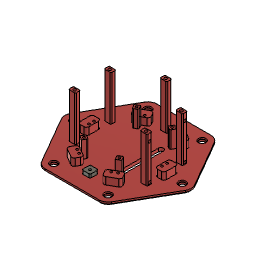
2024-12-28_development_hexapod_mounts (Autodesk Fusion 360 archive; units mm, degrees)
design "base"
Autodesk Fusion 360 part; units mm, degrees
(part 1 of 2)
sketch "Sketch1" plane through (0, 0, 0) normal (0, 0, 1) x (1, 0, 0)
  line L0 (130, 0) -> (65, 112.5833)
  line L1 (65, 112.5833) -> (-65, 112.5833)
  line L2 (-65, 112.5833) -> (-130, 0)
  line L3 (-130, 0) -> (-65, -112.5833)
  line L4 (-65, -112.5833) -> (65, -112.5833)
  line L5 (65, -112.5833) -> (130, 0)
  dimension "d1" = 130
  measures "d1" distance of L0.start origin
extrude "Extrude1" add sketch "Sketch1" along normal blind 6.5 makes body 1
fillet "Fillet1" radius 18 6 edges at (-130, 0, 3.25) (-65, -112.5833, 3.25) (65, -112.5833, 3.25) (130, 0, 3.25) (65, 112.5833, 3.25) (-65, 112.5833, 3.25) on bodies 1
chamfer "Chamfer2" distance 3.25 angle 45 12 edges at (0, -112.5833, 0) (63.6077, -110.1718, 0) (97.5, -56.2917, 0) (127.2154, 0, 0) (97.5, 56.2917, 0) (63.6077, 110.1718, 0) (0, 112.5833, 0) (-63.6077, 110.1718, 0) (-97.5, 56.2917, 0) (-127.2154, 0, 0) (-97.5, -56.2917, 0) (-63.6077, -110.1718, 0) on bodies 1
sketch "Sketch2" plane through (0, 0, 6.5) normal (0, 0, 1) x (-1, 0, 0)
  arc A0 (54.6077, -112.5833) -> (70.1962, -103.5833) centre (54.6077, -94.5833) ccw
  line L0 (70.1962, -103.5833) -> (124.8038, -9)
  arc A1 (124.8038, -9) -> (124.8038, 9) centre (109.2154, 0) ccw
  line L1 (124.8038, 9) -> (70.1962, 103.5833)
  line L2 (54.6077, 112.5833) -> (-54.6077, 112.5833)
  line L3 (-70.1962, 103.5833) -> (-124.8038, 9)
  arc A2 (-124.8038, 9) -> (-124.8038, -9) centre (-109.2154, 0) ccw
  line L4 (-124.8038, -9) -> (-70.1962, -103.5833)
  arc A3 (-70.1962, -103.5833) -> (-54.6077, -112.5833) centre (-54.6077, -94.5833) ccw
  line L5 (-54.6077, -112.5833) -> (54.6077, -112.5833)
  circle A4 centre (109.2154, 0) radius 7
  circle A5 centre (109.2154, 0) radius 6
  circle A6 centre (73.4654, -5) radius 2.25
  arc A7 (73.7154, 14.55) -> (68.7154, 9.55) centre (73.7154, 9.55) ccw
  line L6 (68.7154, 9.55) -> (68.7154, -9.55)
  circle A8 centre (73.4654, 5) radius 2.25
  line L7 (86.7154, 9.55) -> (86.7154, -9.55)
  line L8 (68.7154, 0) -> (86.7154, 0) construction
  arc A9 (68.7154, -9.55) -> (73.7154, -14.55) centre (73.7154, -9.55) ccw
  arc A10 (73.7154, 14.55) -> (68.7154, 9.55) centre (73.7154, 9.55) ccw
  line L9 (81.7154, 14.55) -> (73.7154, 14.55)
  line L10 (73.7154, -14.55) -> (81.7154, -14.55)
  line L11 (73.4654, 5) -> (68.7154, 5) construction
  line L12 (73.4654, -5) -> (68.7154, -5) construction
  line L13 (127.2154, 0) -> (-127.2154, 0) construction
  line L14 (0, -112.5833) -> (0, 112.5833) construction
  arc A11 (-124.8038, 9) -> (-124.8038, -9) centre (-109.2154, 0) ccw
  arc A12 (-70.1962, -103.5833) -> (-54.6077, -112.5833) centre (-54.6077, -94.5833) ccw
  arc A13 (54.6077, -112.5833) -> (70.1962, -103.5833) centre (54.6077, -94.5833) ccw
  arc A14 (81.7154, -14.55) -> (86.7154, -9.55) centre (81.7154, -9.55) ccw
  arc A15 (86.7154, 9.55) -> (81.7154, 14.55) centre (81.7154, 9.55) ccw
  circle A16 centre (32.4026, 66.1229) radius 2.25
  line L15 (34.3577, 59.5093) -> (43.3577, 75.0977) construction
  arc A17 (70.1962, 103.5833) -> (54.6077, 112.5833) centre (54.6077, 94.5833) ccw
  arc A18 (42.6282, 54.7343) -> (49.4584, 56.5644) centre (45.1282, 59.0644) ccw
  line L16 (41.0628, 61.1229) -> (38.6878, 57.0093) construction
  arc A19 (24.257, 71.1144) -> (26.0872, 64.2843) centre (28.5872, 68.6144) ccw
  line L17 (28.257, 78.0426) -> (24.257, 71.1144)
  circle A20 centre (41.0628, 61.1229) radius 2.25
  arc A21 (53.4584, 63.4926) -> (51.6282, 70.3227) centre (49.1282, 65.9926) ccw
  circle A22 centre (54.6077, 94.5833) radius 6
  circle A23 centre (54.6077, 94.5833) radius 7
  line L18 (32.4026, 66.1229) -> (30.0276, 62.0093) construction
  arc A24 (24.257, 71.1144) -> (26.0872, 64.2843) centre (28.5872, 68.6144) ccw
  line L19 (26.0872, 64.2843) -> (42.6282, 54.7343)
  line L20 (49.4584, 56.5644) -> (53.4584, 63.4926)
  line L21 (35.0872, 79.8727) -> (51.6282, 70.3227)
  arc A25 (35.0872, 79.8727) -> (28.257, 78.0426) centre (32.5872, 75.5426) ccw
  circle A26 centre (-41.0628, 61.1229) radius 2.25
  line L22 (-42.6282, 54.7343) -> (-26.0872, 64.2843)
  line L23 (-34.3577, 59.5093) -> (-43.3577, 75.0977) construction
  arc A27 (-54.6077, 112.5833) -> (-70.1962, 103.5833) centre (-54.6077, 94.5833) ccw
  arc A28 (-26.0872, 64.2843) -> (-24.257, 71.1144) centre (-28.5872, 68.6144) ccw
  line L24 (-32.4026, 66.1229) -> (-30.0276, 62.0093) construction
  arc A29 (-49.4584, 56.5644) -> (-42.6282, 54.7343) centre (-45.1282, 59.0644) ccw
  line L25 (-53.4584, 63.4926) -> (-49.4584, 56.5644)
  circle A30 centre (-32.4026, 66.1229) radius 2.25
  arc A31 (-28.257, 78.0426) -> (-35.0872, 79.8727) centre (-32.5872, 75.5426) ccw
  circle A32 centre (-54.6077, 94.5833) radius 6
  circle A33 centre (-54.6077, 94.5833) radius 7
  line L26 (-41.0628, 61.1229) -> (-38.6878, 57.0093) construction
  arc A34 (-49.4584, 56.5644) -> (-42.6282, 54.7343) centre (-45.1282, 59.0644) ccw
  line L27 (-42.6282, 54.7343) -> (-26.0872, 64.2843)
  line L28 (-24.257, 71.1144) -> (-28.257, 78.0426)
  line L29 (-51.6282, 70.3227) -> (-35.0872, 79.8727)
  arc A35 (-51.6282, 70.3227) -> (-53.4584, 63.4926) centre (-49.1282, 65.9926) ccw
  circle A36 centre (-73.4654, -5) radius 2.25
  line L30 (-68.7154, -9.55) -> (-68.7154, 9.55)
  line L31 (-68.7154, 0) -> (-86.7154, 0) construction
  arc A37 (-124.8038, 9) -> (-124.8038, -9) centre (-109.2154, 0) ccw
  arc A38 (-68.7154, 9.55) -> (-73.7154, 14.55) centre (-73.7154, 9.55) ccw
  line L32 (-73.4654, 5) -> (-68.7154, 5) construction
  arc A39 (-73.7154, -14.55) -> (-68.7154, -9.55) centre (-73.7154, -9.55) ccw
  line L33 (-81.7154, -14.55) -> (-73.7154, -14.55)
  circle A40 centre (-73.4654, 5) radius 2.25
  arc A41 (-81.7154, 14.55) -> (-86.7154, 9.55) centre (-81.7154, 9.55) ccw
  circle A42 centre (-109.2154, 0) radius 6
  circle A43 centre (-109.2154, 0) radius 7
  line L34 (-73.4654, -5) -> (-68.7154, -5) construction
  arc A44 (-73.7154, -14.55) -> (-68.7154, -9.55) centre (-73.7154, -9.55) ccw
  line L35 (-68.7154, -9.55) -> (-68.7154, 9.55)
  line L36 (-73.7154, 14.55) -> (-81.7154, 14.55)
  line L37 (-86.7154, -9.55) -> (-86.7154, 9.55)
  arc A45 (-86.7154, -9.55) -> (-81.7154, -14.55) centre (-81.7154, -9.55) ccw
  circle A46 centre (-32.4026, -66.1229) radius 2.25
  line L38 (-26.0872, -64.2843) -> (-42.6282, -54.7343)
  line L39 (-34.3577, -59.5093) -> (-43.3577, -75.0977) construction
  arc A47 (-70.1962, -103.5833) -> (-54.6077, -112.5833) centre (-54.6077, -94.5833) ccw
  arc A48 (-42.6282, -54.7343) -> (-49.4584, -56.5644) centre (-45.1282, -59.0644) ccw
  line L40 (-41.0628, -61.1229) -> (-38.6878, -57.0093) construction
  arc A49 (-24.257, -71.1144) -> (-26.0872, -64.2843) centre (-28.5872, -68.6144) ccw
  line L41 (-28.257, -78.0426) -> (-24.257, -71.1144)
  circle A50 centre (-41.0628, -61.1229) radius 2.25
  arc A51 (-53.4584, -63.4926) -> (-51.6282, -70.3227) centre (-49.1282, -65.9926) ccw
  circle A52 centre (-54.6077, -94.5833) radius 6
  circle A53 centre (-54.6077, -94.5833) radius 7
  line L42 (-32.4026, -66.1229) -> (-30.0276, -62.0093) construction
  arc A54 (-24.257, -71.1144) -> (-26.0872, -64.2843) centre (-28.5872, -68.6144) ccw
  line L43 (-26.0872, -64.2843) -> (-42.6282, -54.7343)
  line L44 (-49.4584, -56.5644) -> (-53.4584, -63.4926)
  line L45 (-35.0872, -79.8727) -> (-51.6282, -70.3227)
  arc A55 (-35.0872, -79.8727) -> (-28.257, -78.0426) centre (-32.5872, -75.5426) ccw
  circle A56 centre (41.0628, -61.1229) radius 2.25
  line L46 (34.3577, -59.5093) -> (43.3577, -75.0977) construction
  arc A57 (54.6077, -112.5833) -> (70.1962, -103.5833) centre (54.6077, -94.5833) ccw
  arc A58 (26.0872, -64.2843) -> (24.257, -71.1144) centre (28.5872, -68.6144) ccw
  line L47 (32.4026, -66.1229) -> (30.0276, -62.0093) construction
  arc A59 (49.4584, -56.5644) -> (42.6282, -54.7343) centre (45.1282, -59.0644) ccw
  line L48 (53.4584, -63.4926) -> (49.4584, -56.5644)
  circle A60 centre (32.4026, -66.1229) radius 2.25
  arc A61 (28.257, -78.0426) -> (35.0872, -79.8727) centre (32.5872, -75.5426) ccw
  circle A62 centre (54.6077, -94.5833) radius 6
  circle A63 centre (54.6077, -94.5833) radius 7
  line L49 (41.0628, -61.1229) -> (38.6878, -57.0093) construction
  arc A64 (49.4584, -56.5644) -> (42.6282, -54.7343) centre (45.1282, -59.0644) ccw
  line L50 (42.6282, -54.7343) -> (26.0872, -64.2843)
  line L51 (24.257, -71.1144) -> (28.257, -78.0426)
  line L52 (51.6282, -70.3227) -> (35.0872, -79.8727)
  arc A65 (51.6282, -70.3227) -> (53.4584, -63.4926) centre (49.1282, -65.9926) ccw
  circle A66 centre (73.4654, -5) radius 2.85
  circle A67 centre (73.4654, 5) radius 2.85
  circle A68 centre (41.0628, 61.1229) radius 2.85
  circle A69 centre (32.4026, 66.1229) radius 2.85
  circle A70 centre (-32.4026, 66.1229) radius 2.85
  circle A71 centre (-41.0628, 61.1229) radius 2.85
  circle A72 centre (-73.4654, 5) radius 2.85
  circle A73 centre (-73.4654, -5) radius 2.85
  circle A74 centre (-41.0628, -61.1229) radius 2.85
  circle A75 centre (-32.4026, -66.1229) radius 2.85
  circle A76 centre (32.4026, -66.1229) radius 2.85
  circle A77 centre (41.0628, -61.1229) radius 2.85
  line L53 (-77, -30.6738) -> (-67, -30.6738)
  line L54 (-65, -32.6738) -> (-65, -38.6134)
  line L55 (-67, -40.6134) -> (-77, -40.6134)
  line L56 (-79, -38.6134) -> (-79, -32.6738)
  line L57 (-77, 40.6096) -> (-67, 40.6096)
  line L58 (-65, 38.6096) -> (-65, 32.6738)
  line L59 (-67, 30.6738) -> (-77, 30.6738)
  line L60 (-79, 32.6738) -> (-79, 38.6096)
  line L61 (-72, -35.5) -> (-72, 13.37) construction
  line L62 (-72, 35.5) -> (-72, 30.8281) construction
  circle A78 centre (-72, 35.5) radius 2.85
  circle A79 centre (-72, -35.5) radius 2.85
  arc A80 (-65, -32.6738) -> (-67, -30.6738) centre (-67, -32.6738) ccw
  arc A81 (-67, -40.6134) -> (-65, -38.6134) centre (-67, -38.6134) ccw
  arc A82 (-77, -30.6738) -> (-79, -32.6738) centre (-77, -32.6738) ccw
  arc A83 (-79, -38.6134) -> (-77, -40.6134) centre (-77, -38.6134) ccw
  arc A84 (-67, 30.6738) -> (-65, 32.6738) centre (-67, 32.6738) ccw
  arc A85 (-65, 38.6096) -> (-67, 40.6096) centre (-67, 38.6096) ccw
  arc A86 (-77, 40.6096) -> (-79, 38.6096) centre (-77, 38.6096) ccw
  arc A87 (-79, 32.6738) -> (-77, 30.6738) centre (-77, 32.6738) ccw
  arc A88 (66.7634, -30.6879) -> (65, -32.6738) centre (67, -32.6738) ccw
  arc A89 (77, -40.6134) -> (79, -38.6134) centre (77, -38.6134) ccw
  line L63 (67, -40.6134) -> (77, -40.6134)
  arc A90 (79, -32.6738) -> (77, -30.6738) centre (77, -32.6738) ccw
  line L64 (79, -38.6134) -> (79, -32.6738)
  line L65 (65, -32.6738) -> (65, -38.6134)
  circle A91 centre (72, -35.5) radius 2.85
  arc A92 (65, -38.6134) -> (67, -40.6134) centre (67, -38.6134) ccw
  arc A93 (79, 38.6096) -> (77, 40.6096) centre (77, 38.6096) ccw
  line L66 (77, 40.6096) -> (67, 40.6096)
  arc A94 (77, 30.6738) -> (79, 32.6738) centre (77, 32.6738) ccw
  arc A95 (67, 40.6096) -> (65, 38.6096) centre (67, 38.6096) ccw
  circle A96 centre (72, 35.5) radius 2.85
  arc A97 (65, 32.6738) -> (66.7634, 30.6879) centre (67, 32.6738) ccw
  line L67 (-24, 37.5) -> (-24, -37.5)
  line L68 (-34, -37.5) -> (-34, 37.5)
  line L69 (-34, 40.2042) -> (-24, -40) construction
  line L70 (-24, 40) -> (-34, -40.2042) construction
  line L71 (68.7154, 0) -> (68.7154, 5) construction
  line L72 (63.7154, -5) -> (68.7154, 5) construction
  line L73 (68.7154, -5) -> (63.7154, 5) construction
  line L74 (-42.6282, -54.7343) -> (-26.0872, -64.2843)
  line L75 (42.6282, 54.7343) -> (26.0872, 64.2843)
  line L76 (-42.6282, 54.7343) -> (-26.0872, 64.2843)
  arc A98 (-34, -37.5) -> (-24, -37.5) centre (-29, -37.5) ccw
  arc A99 (-24, 37.5) -> (-34, 37.5) centre (-29, 37.5) ccw
  line L77 (-6, 84.2496) -> (6.5, 84.2496)
  line L78 (8.5, 82.2496) -> (8.5, 69.7496)
  line L79 (6.5, 67.7496) -> (-6, 67.7496)
  line L80 (-8, 69.7496) -> (-8, 82.2496)
  line L81 (-8, 84.2496) -> (8.5, 67.7496) construction
  line L82 (8.5, 84.2496) -> (-8, 67.7496) construction
  arc A100 (6.5, 67.7496) -> (8.5, 69.7496) centre (6.5, 69.7496) ccw
  arc A101 (8.5, 82.2496) -> (6.5, 84.2496) centre (6.5, 82.2496) ccw
  arc A102 (-6, 84.2496) -> (-8, 82.2496) centre (-6, 82.2496) ccw
  arc A103 (-8, 69.7496) -> (-6, 67.7496) centre (-6, 69.7496) ccw
  circle A104 centre (0.25, 75.9996) radius 2.25
  circle A105 centre (0.25, 75.9996) radius 2.85
  circle A106 centre (0, -76) radius 2.85
  line L83 (-5, -71) -> (5, -71)
  line L84 (7, -73) -> (7, -79)
  line L85 (5, -81) -> (-5, -81)
  line L86 (-7, -79) -> (-7, -73)
  line L87 (-7, -71) -> (7, -81) construction
  line L88 (7, -71) -> (-7, -81) construction
  arc A107 (5, -81) -> (7, -79) centre (5, -79) ccw
  arc A108 (7, -73) -> (5, -71) centre (5, -73) ccw
  arc A109 (-5, -71) -> (-7, -73) centre (-5, -73) ccw
  arc A110 (-7, -79) -> (-5, -81) centre (-5, -79) ccw
  line L89 (77, 30.6738) -> (66.7634, 30.6879)
  line L90 (77, -30.6738) -> (66.7634, -30.6879)
  line L91 (65, 32.6738) -> (65, 38.6096)
  line L92 (79, 32.6738) -> (79, 38.6096)
  line L93 (-35.8962, -47.074) -> (-30.7, -50.074)
  line L94 (-29.968, -52.8061) -> (-33.968, -59.7343)
  line L95 (-33.968, -59.7343) -> (-42.6282, -54.7343)
  line L96 (-42.6282, -54.7343) -> (-38.6282, -47.8061)
  line L97 (-37.6282, -46.074) -> (-33.968, -59.7343) construction
  line L98 (-28.968, -51.074) -> (-42.6282, -54.7343) construction
  line L99 (-24.257, -71.1144) -> (-16.5609, -57.7844) construction
  line L100 (-42.6282, -54.7343) -> (-38.8577, -48.2035) construction
  circle A111 centre (-35.7981, -52.9041) radius 2.25
  arc A112 (-29.968, -52.8061) -> (-30.7, -50.074) centre (-31.7, -51.8061) ccw
  arc A113 (-35.8962, -47.074) -> (-38.6282, -47.8061) centre (-36.8962, -48.8061) ccw
  line L101 (-29.968, 52.8061) -> (-33.968, 59.7343)
  line L102 (-35.8962, 47.074) -> (-30.7, 50.074)
  arc A114 (-30.7, 50.074) -> (-29.968, 52.8061) centre (-31.7, 51.8061) ccw
  arc A115 (-38.6282, 47.8061) -> (-35.8962, 47.074) centre (-36.8962, 48.8061) ccw
  line L103 (-42.6282, 54.7343) -> (-38.6282, 47.8061)
  circle A116 centre (-35.7981, 52.9041) radius 2.25
  line L104 (29.968, 52.8061) -> (33.968, 59.7343)
  arc A117 (29.968, 52.8061) -> (30.7, 50.074) centre (31.7, 51.8061) ccw
  line L105 (35.8962, 47.074) -> (30.7, 50.074)
  arc A118 (35.8962, 47.074) -> (38.6282, 47.8061) centre (36.8962, 48.8061) ccw
  line L106 (42.6282, 54.7343) -> (38.6282, 47.8061)
  circle A119 centre (35.7981, 52.9041) radius 2.25
  line L107 (29.968, -52.8061) -> (33.968, -59.7343)
  arc A120 (30.7, -50.074) -> (29.968, -52.8061) centre (31.7, -51.8061) ccw
  line L108 (35.8962, -47.074) -> (30.7, -50.074)
  arc A121 (38.6282, -47.8061) -> (35.8962, -47.074) centre (36.8962, -48.8061) ccw
  line L109 (42.6282, -54.7343) -> (38.6282, -47.8061)
  circle A122 centre (35.7981, -52.9041) radius 2.25
  point P0 (63.6077, 110.1718)
  point P1 (-63.6077, 110.1718)
  point P2 (-127.2154, 0)
  point P3 (-63.6077, -110.1718)
  point P4 (63.6077, -110.1718)
  point P5 (-72, -35.5)
  point P6 (-72, 35.5)
  point P7 (72, -35.5)
  point P8 (72, -35.5)
  point P9 (72, 35.5)
  point P10 (72, 35.5)
  point P11 (-28.9873, 0)
  point P12 (0, 76)
  point P13 (0, 72)
  point P14 (0.25, 75.9996)
  point P15 (0, -76)
  point P16 (-35.7981, -52.9041)
  point P17 (-35.7981, 52.9041)
  dimension "d8" = 14
  dimension "d9" = 12
  dimension "d10" = 18
  dimension "d11" = 9.55
  dimension "d12" = 9.55
  dimension "d15" = 29.1
  dimension "d30" = 5
  dimension "d33" = 4.5
  dimension "d34" = 4.5
  dimension "d35" = 5.7
  dimension "d36" = 5.7
  dimension "d49" = 72
  dimension "d50" = 5.7
  dimension "d51" = 5.7
  dimension "d53" = 2
  dimension "d75" = 35.5
  dimension "d76" = 35.5
  dimension "d78" = 80
  dimension "d79" = 24
  dimension "d84" = 5
  dimension "d85" = 5
  dimension "d86" = 10
  dimension "d135" = 10
  dimension "d164" = 16.5
  dimension "d165" = 16.5
  dimension "d166" = 2
  dimension "d170" = 76
  dimension "d171" = 4.5
  dimension "d172" = 5.7
  dimension "d173" = 5.7
  dimension "d174" = 76
  dimension "d175" = 14
  dimension "d176" = 10
  dimension "d177" = 2
  dimension "d188" = 7
  dimension "d189" = 7
  dimension "d190" = 10
  dimension "d191" = 10
  dimension "d192" = 4.5
  dimension "d193" = 2
  constraint concentric A1 A4
  constraint concentric A4 A5
  constraint coincident A7.end L6.start
  constraint coincident L6.end A9.start
  constraint coincident A9.end L10.start
  constraint coincident A7.start A10.start
  constraint coincident L8.end L7
  constraint parallel L9 L10
  constraint parallel L6 L7
  constraint coincident A8.centre L11.start
  constraint coincident A6.centre L12.start
  constraint midpoint A1 L13.start
  constraint midpoint A2 P2
  constraint midpoint L5 L14.start
  constraint midpoint L2 L14.end
  constraint collinear L8 L13
  constraint tangent L10 A14
  constraint tangent L7 A14
  constraint tangent L7 A15
  constraint tangent L9 A15
  constraint equal A14 A15
  constraint concentric A6 A66
  constraint horizontal L53
  constraint perpendicular L53 L54
  constraint parallel L53 L55
  constraint parallel L54 L56
  constraint horizontal L57
  constraint perpendicular L57 L58
  constraint parallel L57 L59
  constraint parallel L58 L60
  constraint coincident P5 L61.start
  constraint perpendicular L53 L61
  constraint coincident P6 L62.start
  constraint perpendicular L59 L62
  constraint collinear L61 L62
  constraint tangent L54 A80
  constraint tangent L53 A80
  constraint tangent L55 A81
  constraint tangent L54 A81
  constraint equal A80 A81
  constraint tangent L56 A82
  constraint tangent L53 A82
  constraint equal A80 A82
  constraint tangent L55 A83
  constraint tangent L56 A83
  constraint equal A80 A83
  constraint tangent L59 A84
  constraint tangent L58 A84
  constraint equal A80 A84
  constraint tangent L58 A85
  constraint tangent L57 A85
  constraint equal A80 A85
  constraint tangent L60 A86
  constraint tangent L57 A86
  constraint equal A80 A86
  constraint tangent L60 A87
  constraint tangent L59 A87
  constraint equal A80 A87
  constraint symmetric L14 P5 P8
  constraint symmetric L14 P6 P10
  constraint symmetric L14 A78 A96
  constraint symmetric L14 A79 A91
  constraint symmetric L14 L54.start A88.end
  constraint symmetric L14 A80 A88
  constraint symmetric L14 L55.start L63.start
  constraint symmetric L14 L54.end L65.end
  constraint symmetric L14 A81 A92
  constraint symmetric L14 L56.end A90.start
  constraint symmetric L14 L53.start A90.end
  constraint symmetric L14 A82 A90
  constraint symmetric L14 L55.end A89.start
  constraint symmetric L14 L56.start A89.end
  constraint symmetric L14 A83 A89
  constraint symmetric L14 L58.end A97.start
  constraint symmetric L14 A84 A97
  constraint symmetric L14 L58.start A95.end
  constraint symmetric L14 L57.end L66.end
  constraint symmetric L14 A85 A95
  constraint symmetric L14 L60.end A93.start
  constraint symmetric L14 L57.start A93.end
  constraint symmetric L14 A86 A93
  constraint symmetric L14 L60.start A94.end
  constraint symmetric L14 L59.end A94.start
  constraint symmetric L14 A87 A94
  constraint parallel L67 L68
  constraint coincident L69 P11
  constraint coincident L70 P11
  constraint coincident L13 P11
  constraint coincident L69.end L67
  constraint coincident L70.end L68
  constraint coincident L70.start L67
  constraint coincident L69.start L68
  constraint perpendicular L8 L71
  constraint symmetric L14 A58.start L38.start
  constraint symmetric L14 A59.end L38.end
  constraint symmetric L13 A58.start A19.end
  constraint symmetric L13 L38.start L22.end
  constraint tangent L68 A98
  constraint tangent L68 A99
  constraint horizontal L77
  constraint perpendicular L77 L78
  constraint parallel L77 L79
  constraint parallel L78 L80
  constraint coincident L81 P14
  constraint coincident L82 P14
  constraint coincident L81.end L79
  constraint coincident L81.end L78
  constraint tangent L79 A100
  constraint tangent L78 A100
  constraint coincident L82.start L78
  constraint coincident L82.start L77
  constraint tangent L78 A101
  constraint tangent L77 A101
  constraint equal A100 A101
  constraint coincident L81.start L77
  constraint coincident L81.start L80
  constraint tangent L77 A102
  constraint tangent L80 A102
  constraint equal A100 A102
  constraint coincident L82.end L80
  constraint coincident L82.end L79
  constraint tangent L80 A103
  constraint tangent L79 A103
  constraint equal A100 A103
  constraint coincident P14 A104.centre
  constraint concentric A104 A105
  constraint coincident L14 P15
  constraint horizontal L83
  constraint perpendicular L83 L84
  constraint parallel L83 L85
  constraint parallel L84 L86
  constraint coincident L87 P15
  constraint coincident L88 P15
  constraint coincident P15 A106.centre
  constraint coincident L87.end L85
  constraint coincident L87.end L84
  constraint tangent L85 A107
  constraint tangent L84 A107
  constraint coincident L88.start L84
  constraint coincident L88.start L83
  constraint tangent L84 A108
  constraint tangent L83 A108
  constraint equal A107 A108
  constraint coincident L87.start L83
  constraint coincident L87.start L86
  constraint tangent L83 A109
  constraint tangent L86 A109
  constraint equal A107 A109
  constraint coincident L88.end L86
  constraint coincident L88.end L85
  constraint tangent L86 A110
  constraint tangent L85 A110
  constraint equal A107 A110
  constraint tangent A93 L92
  constraint perpendicular L93 L94
  constraint parallel L93 L95
  constraint parallel L94 L96
  constraint coincident L97 P16
  constraint coincident L98 P16
  constraint collinear L43 L95
  constraint tangent A54 L99
  constraint parallel L41 L99
  constraint perpendicular L43 L100
  constraint collinear L96 L100
  constraint coincident P16 A111.centre
  constraint coincident L98.start L94
  constraint coincident L98.start L93
  constraint tangent L94 A112
  constraint tangent L93 A112
  constraint coincident L97.start L93
  constraint coincident L97.start L96
  constraint tangent L93 A113
  constraint tangent L96 A113
  constraint equal A112 A113
  constraint symmetric L13 L94.end L101.end
  constraint symmetric L13 L38.end L22.start
  constraint symmetric L13 P16 P17
  constraint symmetric L13 A111 A116
  constraint symmetric L13 L94.start L101.start
  constraint symmetric L13 L93.end L102.end
  constraint symmetric L13 A112 A114
  constraint symmetric L13 L93.start L102.start
  constraint symmetric L13 L96.end A115.start
  constraint symmetric L13 A113 A115
  constraint symmetric L14 L94.end L107.end
  constraint symmetric L14 L38.end A59.end
  constraint symmetric L14 A111 A122
  constraint symmetric L14 L94.start L107.start
  constraint symmetric L14 L93.end A120.start
  constraint symmetric L14 A112 A120
  constraint symmetric L14 L93.start L108.start
  constraint symmetric L14 L96.end A121.start
  constraint symmetric L14 A113 A121
  constraint symmetric L14 L101.start L104.start
  constraint symmetric L14 L101.end L104.end
  constraint symmetric L14 L102.start L105.start
  constraint symmetric L14 L102.end A117.end
  constraint symmetric L14 A114 A117
  constraint symmetric L14 A115.start A118.end
  constraint symmetric L14 A115 A118
  constraint symmetric L14 L22.start A18.start
  constraint symmetric L14 A116 A119
  measures "d8" diameter of A4
  measures "d9" diameter of A5
  measures "d10" distance of L8.end L8.start
  measures "d11" distance of A8.centre L9
  measures "d12" distance of A6.centre L10
  measures "d15" distance of L9 L10
  measures "d30" radius of A14
  measures "d33" diameter of A6
  measures "d34" diameter of A8
  measures "d35" diameter of A66
  measures "d36" diameter of A67
  measures "d49" distance of L14 P6
  measures "d50" diameter of A78
  measures "d51" diameter of A79
  measures "d53" radius of A80
  measures "d75" distance of L13 P5
  measures "d76" distance of L13 P6
  measures "d78" distance of L70.start L69.end
  measures "d79" distance of origin L67
  measures "d84" distance of L8.start L11.end
  measures "d85" distance of L11.end L73.end
  measures "d86" distance of L11.end L12.end
  measures "d135" distance of L67 L68
  measures "d164" distance of L81.end L82.end
  measures "d165" distance of L82.start L81.end
  measures "d166" radius of A100
  measures "d170" distance of origin P14
  measures "d171" diameter of A104
  measures "d172" diameter of A105
  measures "d173" diameter of A106
  measures "d174" distance of origin P15
  measures "d175" distance of L87.end L88.end
  measures "d176" distance of L88.start L87.end
  measures "d177" radius of A107
  measures "d188" distance of P8 L64
  measures "d189" distance of P8 L65
  measures "d190" distance of L94.end L38.end
  measures "d191" distance of L98.start L94.end
  measures "d192" diameter of A111
  measures "d193" radius of A112
extrude "Extrude2" cut sketch "Sketch2" against normal blind 6.5 contours A5 | A22 | A32 | A42 | A52 | A62 bodies 1
extrude "Extrude3" cut sketch "Sketch2" along normal blind 4.25 from surface at -6.5 contours A4 | A23 | A33 | A43 | A53 | A63 bodies 1
fillet "Fillet5" radius 0.5 6 edges at (-102.6891, 2.5313, 4.25) (-53.5367, -87.6657, 4.25) (49.1524, -90.197, 4.25) (-49.1524, 90.197, 4.25) (53.5367, 87.6657, 4.25) (102.6891, -2.5313, 4.25) on bodies 1
chamfer "Chamfer1" distance 1.5 angle 45 6 edges at (-103.6214, -2.1697, 6.5) (-53.6897, 88.6539, 6.5) (-49.9317, -90.8236, 6.5) (53.6897, -88.6539, 6.5) (49.9317, 90.8236, 6.5) (103.6214, 2.1697, 6.5) on bodies 1
extrude "Extrude4" add sketch "Sketch2" along normal blind 14.5 contours A7 L6 L7 A9 A10 L9 L10 A14 A15 | A18 A19 L17 A21 A24 L19 L20 L21 A25 L75 | L22 A28 A29 L25 A31 A34 L27 L28 L29 A35 L76 | L30 A38 A39 L33 A41 A44 L35 L36 L37 A45 | L38 A48 A49 L41 A51 A54 L43 L44 L45 A55 L74 L95 | A58 A59 L48 A61 A64 L50 L51 L52 A65 | A66 | A67 | A68 | A69 | A70 | A71 | A72 | A73 | A74 | A75 | A76 | A77 bodies 1
extrude "Extrude6" cut sketch "Sketch2" against normal blind 6.5 contours A6 | A8 | A16 | A20 | A26 | A30 | A36 | A40 | A46 | A50 | A56 | A60 | A66 | A67 | A68 | A69 | A70 | A71 | A72 | A73 | A74 | A75 | A76 | A77 bodies 1
extrude "Extrude25" add sketch "Sketch2" along normal blind 34 contours L19 L75 L104 A117 L105 A118 L106 | L22 L27 L76 L101 L102 A114 A115 L103 | L38 L43 L74 L93 L94 L95 L96 A112 A113 | L50 L107 A120 L108 A121 L109 | A111 | A116 | A119 | A122 bodies 1
extrude "Extrude26" cut sketch "Sketch2" against normal blind 5 from surface at 34 contours A111 | A116 | A119 | A122 bodies 1
extrude "Extrude7" add sketch "Sketch2" along normal blind 90 contours L53 L54 L55 L56 A80 A81 A82 A83 | L57 L58 L59 L60 A84 A85 A86 A87 | A78 | A79 | A88 A89 L63 A90 L64 L65 A92 L90 | A91 | A93 L66 A94 A95 A97 L89 L91 L92 | A96 | A106 | L83 L84 L85 L86 A107 A108 A109 A110 bodies 1
extrude "Extrude8" cut sketch "Sketch2" against normal blind 5 from surface at 90 contours A78 | A79 | A91 | A96 | A106 bodies 1
extrude "Extrude20" add sketch "Sketch2" along normal blind 7 separate body contours L77 L78 L79 L80 A100 A101 A102 A103 | A105 makes body 2
extrude "Extrude21" cut sketch "Sketch2" against normal blind 6.5 from surface at -1.5 contours A104 | A105 bodies 1
extrude "Extrude22" cut sketch "Sketch2" against normal blind 6.5 contours A104 bodies 1
sketch "Sketch4" plane through (79, 0, 0) normal (1, 0, 0) x (0, 1, 0)
  line L0 (32.6738, 6.5) -> (38.6134, 6.5)
  line L1 (38.6134, 6.5) -> (38.6134, 96.5)
  line L2 (38.6134, 96.5) -> (32.6738, 96.5)
  line L3 (32.6738, 96.5) -> (32.6738, 6.5)
  circle A0 centre (-35.6417, 82.5) radius 2.75
  circle A1 centre (-35.6417, 82.5) radius 1.75
  line L4 (-32.6738, 6.5) -> (-38.6096, 6.5) construction
  line L5 (38.6134, 6.5) -> (32.6738, 6.5) construction
  line L6 (-35.6417, 6.5) -> (-35.6417, 81) construction
  line L7 (-35.6417, 82.5) -> (-35.6417, 79.75) construction
  circle A2 centre (-35.6417, 10.5) radius 2.75
  circle A3 centre (-35.6417, 10.5) radius 1.75
  line L8 (0, 2.5) -> (0, 20) construction
  circle A4 centre (35.6417, 10.5) radius 1.75
  circle A5 centre (35.6417, 10.5) radius 2.75
  circle A6 centre (35.6417, 82.5) radius 1.75
  line L9 (35.6417, 6.5) -> (35.6417, 81) construction
  line L10 (32.6738, 6.5) -> (38.6096, 6.5) construction
  line L11 (35.6417, 82.5) -> (35.6417, 79.75) construction
  circle A7 centre (35.6417, 82.5) radius 2.75
  dimension "d59" = 5.5
  dimension "d60" = 3.5
  dimension "d62" = 76
  dimension "d63" = 5.5
  dimension "d64" = 4
  dimension "d65" = 3.5
  constraint concentric A0 A1
  constraint midpoint L4 L6.start
  constraint perpendicular L4 L6
  constraint coincident A0.centre A1.centre
  constraint coincident A0 L7.end
  constraint vertical L7
  constraint collinear L6 L7
  constraint coincident L6 A2.centre
  constraint concentric A2 A3
  constraint symmetric A0 L8 A7
  constraint symmetric A1 L8 A6
  constraint symmetric L4.start L8 L0.start
  constraint symmetric L4.end L8 L10.end
  constraint symmetric L6.start L8 L9.start
  constraint symmetric L6.end L8 L9.end
  constraint symmetric A0.centre L8 A6.centre
  constraint symmetric L7.end L8 L11.end
  constraint symmetric A2 L8 A5
  constraint symmetric A3 L8 A4
  measures "d59" diameter of A0
  measures "d60" diameter of A1
  measures "d62" distance of A0.centre L6.start
  measures "d63" diameter of A2
  measures "d64" distance of L4 A2.centre
  measures "d65" diameter of A3
extrude "Extrude9" cut sketch "Sketch4" against normal blind 5 contours A0 | A1 | A2 | A3 | A4 | A5 | A6 | A7 bodies 1
extrude "Extrude10" cut sketch "Sketch4" against normal up to surface (14 mm away) contours A1 | A3 | A4 | A6 bodies 1
extrude "Extrude11" cut sketch "Sketch2" against normal blind 6.5 contours L67 L68 A98 A99 bodies 1
sketch "Sketch6" plane through (0, 0, 0) normal (0, 0, -1) x (1, 0, 0)
  line L0 (34, 37.5) -> (34, -37.5)
  line L1 (24, -37.5) -> (24, 37.5)
  circle A0 centre (109.2154, 0) radius 7
  circle A1 centre (-109.2154, 0) radius 7
  circle A2 centre (54.6077, 94.5833) radius 7
  circle A3 centre (54.6077, -94.5833) radius 7
  circle A4 centre (-54.6077, -94.5833) radius 7
  circle A5 centre (-54.6077, 94.5833) radius 7
  line L2 (54.6077, 109.3333) -> (-54.6077, 109.3333)
  arc A6 (-54.6077, 109.3333) -> (-67.3816, 101.9583) centre (-54.6077, 94.5833) ccw
  line L3 (-67.3816, 101.9583) -> (-121.9893, 7.375)
  arc A7 (-121.9893, 7.375) -> (-121.9893, -7.375) centre (-109.2154, 0) ccw
  line L4 (-121.9893, -7.375) -> (-67.3816, -101.9583)
  arc A8 (-67.3816, -101.9583) -> (-54.6077, -109.3333) centre (-54.6077, -94.5833) ccw
  line L5 (-54.6077, -109.3333) -> (54.6077, -109.3333)
  arc A9 (54.6077, -109.3333) -> (67.3816, -101.9583) centre (54.6077, -94.5833) ccw
  line L6 (67.3816, -101.9583) -> (121.9893, -7.375)
  arc A10 (121.9893, -7.375) -> (121.9893, 7.375) centre (109.2154, 0) ccw
  line L7 (121.9893, 7.375) -> (67.3816, 101.9583)
  arc A11 (67.3816, 101.9583) -> (54.6077, 109.3333) centre (54.6077, 94.5833) ccw
  line L8 (0, 0) -> (-123.9654, 0) construction
  circle A12 centre (-89.2154, 0) radius 2.35
  line L9 (-53.7561, -78.4378) -> (-50.1995, -84.598)
  arc A13 (-48.1643, -68.6025) -> (-50.3294, -69.8525) centre (-48.1643, -71.1025) ccw
  line L10 (-39.0159, -84.598) -> (-35.4593, -78.4378)
  arc A14 (-41.0511, -85.923) -> (-38.886, -84.673) centre (-41.0511, -83.423) ccw
  line L11 (-48.1643, -85.923) -> (-41.0511, -85.923)
  arc A15 (-53.7561, -76.0878) -> (-53.7561, -78.4378) centre (-51.7209, -77.2628) ccw
  arc A16 (-41.0511, -85.773) -> (-39.0159, -84.598) centre (-41.0511, -83.423) ccw
  line L12 (-41.0511, -68.7525) -> (-48.1643, -68.7525)
  line L13 (-53.886, -78.5128) -> (-50.3294, -84.673)
  line L14 (-35.3294, -76.0128) -> (-38.886, -69.8525)
  arc A17 (-35.3294, -78.5128) -> (-35.3294, -76.0128) centre (-37.4944, -77.2628) ccw
  arc A18 (-38.886, -69.8525) -> (-41.0511, -68.6025) centre (-41.0511, -71.1025) ccw
  circle A19 centre (-32.4026, -66.1229) radius 2.85
  line L15 (-35.4593, -76.0878) -> (-39.0159, -69.9275)
  line L16 (-48.1643, -85.773) -> (-41.0511, -85.773)
  circle A20 centre (-44.6077, -77.2628) radius 2.35
  arc A21 (-35.4593, -78.4378) -> (-35.4593, -76.0878) centre (-37.4944, -77.2628) ccw
  arc A22 (-50.3294, -84.673) -> (-48.1643, -85.923) centre (-48.1643, -83.423) ccw
  arc A23 (-53.886, -76.0128) -> (-53.886, -78.5128) centre (-51.7209, -77.2628) ccw
  line L17 (-38.886, -84.673) -> (-35.3294, -78.5128)
  line L18 (-50.1995, -69.9275) -> (-53.7561, -76.0878)
  arc A24 (-39.0159, -69.9275) -> (-41.0511, -68.7525) centre (-41.0511, -71.1025) ccw
  arc A25 (-48.1643, -68.7525) -> (-50.1995, -69.9275) centre (-48.1643, -71.1025) ccw
  line L19 (-50.3294, -69.8525) -> (-53.886, -76.0128)
  line L20 (-41.0511, -68.6025) -> (-48.1643, -68.6025)
  arc A26 (-50.1995, -84.598) -> (-48.1643, -85.773) centre (-48.1643, -83.423) ccw
  circle A27 centre (-41.0628, -61.1229) radius 2.85
  line L21 (41.0511, -85.773) -> (48.1643, -85.773)
  arc A28 (35.3294, -76.0128) -> (35.3294, -78.5128) centre (37.4944, -77.2628) ccw
  line L22 (53.7561, -76.0878) -> (50.1995, -69.9275)
  arc A29 (53.886, -78.5128) -> (53.886, -76.0128) centre (51.7209, -77.2628) ccw
  line L23 (50.3294, -84.673) -> (53.886, -78.5128)
  arc A30 (39.0159, -84.598) -> (41.0511, -85.773) centre (41.0511, -83.423) ccw
  arc A31 (53.7561, -78.4378) -> (53.7561, -76.0878) centre (51.7209, -77.2628) ccw
  line L24 (39.0159, -69.9275) -> (35.4593, -76.0878)
  line L25 (41.0511, -85.923) -> (48.1643, -85.923)
  line L26 (48.1643, -68.6025) -> (41.0511, -68.6025)
  arc A32 (50.3294, -69.8525) -> (48.1643, -68.6025) centre (48.1643, -71.1025) ccw
  arc A33 (41.0511, -68.6025) -> (38.886, -69.8525) centre (41.0511, -71.1025) ccw
  circle A34 centre (41.0628, -61.1229) radius 2.85
  line L27 (48.1643, -68.7525) -> (41.0511, -68.7525)
  line L28 (50.1995, -84.598) -> (53.7561, -78.4378)
  circle A35 centre (44.6077, -77.2628) radius 2.35
  arc A36 (50.1995, -69.9275) -> (48.1643, -68.7525) centre (48.1643, -71.1025) ccw
  arc A37 (48.1643, -85.923) -> (50.3294, -84.673) centre (48.1643, -83.423) ccw
  arc A38 (38.886, -84.673) -> (41.0511, -85.923) centre (41.0511, -83.423) ccw
  line L29 (53.886, -76.0128) -> (50.3294, -69.8525)
  line L30 (35.4593, -78.4378) -> (39.0159, -84.598)
  arc A39 (41.0511, -68.7525) -> (39.0159, -69.9275) centre (41.0511, -71.1025) ccw
  arc A40 (35.4593, -76.0878) -> (35.4593, -78.4378) centre (37.4944, -77.2628) ccw
  line L31 (35.3294, -78.5128) -> (38.886, -84.673)
  line L32 (38.886, -69.8525) -> (35.3294, -76.0128)
  arc A41 (48.1643, -85.773) -> (50.1995, -84.598) centre (48.1643, -83.423) ccw
  circle A42 centre (32.4026, -66.1229) radius 2.85
  line L33 (94.8072, -7.3353) -> (98.3638, -1.175)
  arc A43 (83.4937, -7.4103) -> (85.6588, -8.6603) centre (85.6588, -6.1603) ccw
  line L34 (92.772, 8.5103) -> (85.6588, 8.5103)
  arc A44 (94.9371, 7.4103) -> (92.772, 8.6603) centre (92.772, 6.1603) ccw
  line L35 (98.4937, 1.25) -> (94.9371, 7.4103)
  arc A45 (92.772, -8.5103) -> (94.8072, -7.3353) centre (92.772, -6.1603) ccw
  arc A46 (94.8072, 7.3353) -> (92.772, 8.5103) centre (92.772, 6.1603) ccw
  line L36 (80.067, -1.175) -> (83.6236, -7.3353)
  line L37 (94.9371, -7.4103) -> (98.4937, -1.25)
  line L38 (83.4937, 7.4103) -> (79.9371, 1.25)
  arc A47 (85.6588, 8.6603) -> (83.4937, 7.4103) centre (85.6588, 6.1603) ccw
  arc A48 (79.9371, 1.25) -> (79.9371, -1.25) centre (82.1021, 0) ccw
  circle A49 centre (73.4654, 5) radius 2.85
  line L39 (83.6236, 7.3353) -> (80.067, 1.175)
  line L40 (98.3638, 1.175) -> (94.8072, 7.3353)
  circle A50 centre (89.2154, 0) radius 2.35
  arc A51 (85.6588, 8.5103) -> (83.6236, 7.3353) centre (85.6588, 6.1603) ccw
  arc A52 (98.4937, -1.25) -> (98.4937, 1.25) centre (96.3286, 0) ccw
  arc A53 (92.772, -8.6603) -> (94.9371, -7.4103) centre (92.772, -6.1603) ccw
  line L41 (92.772, 8.6603) -> (85.6588, 8.6603)
  line L42 (85.6588, -8.5103) -> (92.772, -8.5103)
  arc A54 (80.067, 1.175) -> (80.067, -1.175) centre (82.1021, 0) ccw
  arc A55 (83.6236, -7.3353) -> (85.6588, -8.5103) centre (85.6588, -6.1603) ccw
  line L43 (85.6588, -8.6603) -> (92.772, -8.6603)
  line L44 (79.9371, -1.25) -> (83.4937, -7.4103)
  arc A56 (98.3638, -1.175) -> (98.3638, 1.175) centre (96.3286, 0) ccw
  circle A57 centre (73.4654, -5) radius 2.85
  line L45 (53.7561, 78.4378) -> (50.1995, 84.598)
  arc A58 (48.1643, 68.6025) -> (50.3294, 69.8525) centre (48.1643, 71.1025) ccw
  line L46 (39.0159, 84.598) -> (35.4593, 78.4378)
  arc A59 (41.0511, 85.923) -> (38.886, 84.673) centre (41.0511, 83.423) ccw
  line L47 (48.1643, 85.923) -> (41.0511, 85.923)
  arc A60 (53.7561, 76.0878) -> (53.7561, 78.4378) centre (51.7209, 77.2628) ccw
  arc A61 (41.0511, 85.773) -> (39.0159, 84.598) centre (41.0511, 83.423) ccw
  line L48 (41.0511, 68.7525) -> (48.1643, 68.7525)
  line L49 (53.886, 78.5128) -> (50.3294, 84.673)
  line L50 (35.3294, 76.0128) -> (38.886, 69.8525)
  arc A62 (35.3294, 78.5128) -> (35.3294, 76.0128) centre (37.4944, 77.2628) ccw
  arc A63 (38.886, 69.8525) -> (41.0511, 68.6025) centre (41.0511, 71.1025) ccw
  circle A64 centre (32.4026, 66.1229) radius 2.85
  line L51 (35.4593, 76.0878) -> (39.0159, 69.9275)
  line L52 (48.1643, 85.773) -> (41.0511, 85.773)
  circle A65 centre (44.6077, 77.2628) radius 2.35
  arc A66 (35.4593, 78.4378) -> (35.4593, 76.0878) centre (37.4944, 77.2628) ccw
  arc A67 (50.3294, 84.673) -> (48.1643, 85.923) centre (48.1643, 83.423) ccw
  arc A68 (53.886, 76.0128) -> (53.886, 78.5128) centre (51.7209, 77.2628) ccw
  line L53 (38.886, 84.673) -> (35.3294, 78.5128)
  line L54 (50.1995, 69.9275) -> (53.7561, 76.0878)
  arc A69 (39.0159, 69.9275) -> (41.0511, 68.7525) centre (41.0511, 71.1025) ccw
  arc A70 (48.1643, 68.7525) -> (50.1995, 69.9275) centre (48.1643, 71.1025) ccw
  line L55 (50.3294, 69.8525) -> (53.886, 76.0128)
  line L56 (41.0511, 68.6025) -> (48.1643, 68.6025)
  arc A71 (50.1995, 84.598) -> (48.1643, 85.773) centre (48.1643, 83.423) ccw
  circle A72 centre (41.0628, 61.1229) radius 2.85
  line L57 (-41.0511, 85.773) -> (-48.1643, 85.773)
  arc A73 (-35.3294, 76.0128) -> (-35.3294, 78.5128) centre (-37.4944, 77.2628) ccw
  line L58 (-53.7561, 76.0878) -> (-50.1995, 69.9275)
  arc A74 (-53.886, 78.5128) -> (-53.886, 76.0128) centre (-51.7209, 77.2628) ccw
  line L59 (-50.3294, 84.673) -> (-53.886, 78.5128)
  arc A75 (-39.0159, 84.598) -> (-41.0511, 85.773) centre (-41.0511, 83.423) ccw
  arc A76 (-53.7561, 78.4378) -> (-53.7561, 76.0878) centre (-51.7209, 77.2628) ccw
  line L60 (-39.0159, 69.9275) -> (-35.4593, 76.0878)
  line L61 (-41.0511, 85.923) -> (-48.1643, 85.923)
  line L62 (-48.1643, 68.6025) -> (-41.0511, 68.6025)
  arc A77 (-50.3294, 69.8525) -> (-48.1643, 68.6025) centre (-48.1643, 71.1025) ccw
  arc A78 (-41.0511, 68.6025) -> (-38.886, 69.8525) centre (-41.0511, 71.1025) ccw
  circle A79 centre (-41.0628, 61.1229) radius 2.85
  line L63 (-48.1643, 68.7525) -> (-41.0511, 68.7525)
  line L64 (-50.1995, 84.598) -> (-53.7561, 78.4378)
  circle A80 centre (-44.6077, 77.2628) radius 2.35
  arc A81 (-50.1995, 69.9275) -> (-48.1643, 68.7525) centre (-48.1643, 71.1025) ccw
  arc A82 (-48.1643, 85.923) -> (-50.3294, 84.673) centre (-48.1643, 83.423) ccw
  arc A83 (-38.886, 84.673) -> (-41.0511, 85.923) centre (-41.0511, 83.423) ccw
  line L65 (-53.886, 76.0128) -> (-50.3294, 69.8525)
  line L66 (-35.4593, 78.4378) -> (-39.0159, 84.598)
  arc A84 (-41.0511, 68.7525) -> (-39.0159, 69.9275) centre (-41.0511, 71.1025) ccw
  arc A85 (-35.4593, 76.0878) -> (-35.4593, 78.4378) centre (-37.4944, 77.2628) ccw
  line L67 (-35.3294, 78.5128) -> (-38.886, 84.673)
  line L68 (-38.886, 69.8525) -> (-35.3294, 76.0128)
  arc A86 (-48.1643, 85.773) -> (-50.1995, 84.598) centre (-48.1643, 83.423) ccw
  circle A87 centre (-32.4026, 66.1229) radius 2.85
  circle A88 centre (-89.2154, 0) radius 1.75
  circle A89 centre (0, 0) radius 1.5
  line L69 (-93.947, 8.1954) -> (-84.4838, -8.1954) construction
  line L70 (-84.4838, 8.1954) -> (-93.947, -8.1954) construction
  line L71 (-98.0607, -1) -> (-94.5041, -7.1603)
  arc A90 (-94.5041, -7.1603) -> (-92.772, -8.1603) centre (-92.772, -6.1603) ccw
  line L72 (-92.772, -8.1603) -> (-85.6588, -8.1603)
  arc A91 (-85.6588, -8.1603) -> (-83.9267, -7.1603) centre (-85.6588, -6.1603) ccw
  line L73 (-83.9267, -7.1603) -> (-80.3701, -1)
  arc A92 (-80.3701, -1) -> (-80.3701, 1) centre (-82.1021, 0) ccw
  line L74 (-80.3701, 1) -> (-83.9267, 7.1603)
  arc A93 (-83.9267, 7.1603) -> (-85.6588, 8.1603) centre (-85.6588, 6.1603) ccw
  line L75 (-85.6588, 8.1603) -> (-92.772, 8.1603)
  arc A94 (-92.772, 8.1603) -> (-94.5041, 7.1603) centre (-92.772, 6.1603) ccw
  line L76 (-94.5041, 7.1603) -> (-98.0607, 1)
  arc A95 (-98.0607, 1) -> (-98.0607, -1) centre (-96.3286, 0) ccw
  arc A96 (34, 37.5) -> (24, 37.5) centre (29, 37.5) ccw
  arc A97 (24, -37.5) -> (34, -37.5) centre (29, -37.5) ccw
  circle A98 centre (73.4654, 5) radius 2.85
  circle A99 centre (-32.4026, -66.1229) radius 2.85
  circle A100 centre (-73.4654, -5) radius 2.85
  circle A101 centre (-41.0628, 61.1229) radius 2.85
  circle A102 centre (32.4026, -66.1229) radius 2.85
  circle A103 centre (41.0628, 61.1229) radius 2.85
  circle A104 centre (73.4654, -5) radius 2.85
  circle A105 centre (-41.0628, -61.1229) radius 2.85
  circle A106 centre (-73.4654, 5) radius 2.85
  circle A107 centre (-32.4026, 66.1229) radius 2.85
  circle A108 centre (41.0628, -61.1229) radius 2.85
  circle A109 centre (32.4026, 66.1229) radius 2.85
  line L77 (-94.9371, 7.4103) -> (-98.4937, 1.25)
  arc A110 (-98.4937, 1.25) -> (-98.4937, -1.25) centre (-96.3286, 0) ccw
  line L78 (-98.4937, -1.25) -> (-94.9371, -7.4103)
  arc A111 (-94.9371, -7.4103) -> (-92.772, -8.6603) centre (-92.772, -6.1603) ccw
  line L79 (-92.772, -8.6603) -> (-85.6588, -8.6603)
  arc A112 (-85.6588, -8.6603) -> (-83.4937, -7.4103) centre (-85.6588, -6.1603) ccw
  line L80 (-83.4937, -7.4103) -> (-79.9371, -1.25)
  arc A113 (-79.9371, -1.25) -> (-79.9371, 1.25) centre (-82.1021, 0) ccw
  line L81 (-79.9371, 1.25) -> (-83.4937, 7.4103)
  arc A114 (-83.4937, 7.4103) -> (-85.6588, 8.6603) centre (-85.6588, 6.1603) ccw
  line L82 (-85.6588, 8.6603) -> (-92.772, 8.6603)
  arc A115 (-92.772, 8.6603) -> (-94.9371, 7.4103) centre (-92.772, 6.1603) ccw
  arc A116 (-50.3294, -84.673) -> (-48.1643, -85.923) centre (-48.1643, -83.423) ccw
  line L83 (-48.1643, -85.923) -> (-41.0511, -85.923)
  arc A117 (-41.0511, -85.923) -> (-38.886, -84.673) centre (-41.0511, -83.423) ccw
  line L84 (-38.886, -84.673) -> (-35.3294, -78.5128)
  arc A118 (-35.3294, -78.5128) -> (-35.3294, -76.0128) centre (-37.4944, -77.2628) ccw
  line L85 (-35.3294, -76.0128) -> (-38.886, -69.8525)
  arc A119 (-38.886, -69.8525) -> (-41.0511, -68.6025) centre (-41.0511, -71.1025) ccw
  line L86 (-41.0511, -68.6025) -> (-48.1643, -68.6025)
  arc A120 (-48.1643, -68.6025) -> (-50.3294, -69.8525) centre (-48.1643, -71.1025) ccw
  line L87 (-53.886, -78.5128) -> (-50.3294, -84.673)
  arc A121 (-53.886, -76.0128) -> (-53.886, -78.5128) centre (-51.7209, -77.2628) ccw
  line L88 (-50.3294, -69.8525) -> (-53.886, -76.0128)
  arc A122 (48.1643, -85.923) -> (50.3294, -84.673) centre (48.1643, -83.423) ccw
  line L89 (50.3294, -84.673) -> (53.886, -78.5128)
  arc A123 (53.886, -78.5128) -> (53.886, -76.0128) centre (51.7209, -77.2628) ccw
  line L90 (53.886, -76.0128) -> (50.3294, -69.8525)
  arc A124 (50.3294, -69.8525) -> (48.1643, -68.6025) centre (48.1643, -71.1025) ccw
  line L91 (48.1643, -68.6025) -> (41.0511, -68.6025)
  arc A125 (41.0511, -68.6025) -> (38.886, -69.8525) centre (41.0511, -71.1025) ccw
  line L92 (38.886, -69.8525) -> (35.3294, -76.0128)
  arc A126 (35.3294, -76.0128) -> (35.3294, -78.5128) centre (37.4944, -77.2628) ccw
  line L93 (41.0511, -85.923) -> (48.1643, -85.923)
  arc A127 (38.886, -84.673) -> (41.0511, -85.923) centre (41.0511, -83.423) ccw
  line L94 (35.3294, -78.5128) -> (38.886, -84.673)
  arc A128 (98.4937, -1.25) -> (98.4937, 1.25) centre (96.3286, 0) ccw
  line L95 (98.4937, 1.25) -> (94.9371, 7.4103)
  arc A129 (94.9371, 7.4103) -> (92.772, 8.6603) centre (92.772, 6.1603) ccw
  line L96 (92.772, 8.6603) -> (85.6588, 8.6603)
  arc A130 (85.6588, 8.6603) -> (83.4937, 7.4103) centre (85.6588, 6.1603) ccw
  line L97 (83.4937, 7.4103) -> (79.9371, 1.25)
  arc A131 (79.9371, 1.25) -> (79.9371, -1.25) centre (82.1021, 0) ccw
  line L98 (79.9371, -1.25) -> (83.4937, -7.4103)
  arc A132 (83.4937, -7.4103) -> (85.6588, -8.6603) centre (85.6588, -6.1603) ccw
  line L99 (94.9371, -7.4103) -> (98.4937, -1.25)
  arc A133 (92.772, -8.6603) -> (94.9371, -7.4103) centre (92.772, -6.1603) ccw
  line L100 (85.6588, -8.6603) -> (92.772, -8.6603)
  arc A134 (50.3294, 84.673) -> (48.1643, 85.923) centre (48.1643, 83.423) ccw
  line L101 (48.1643, 85.923) -> (41.0511, 85.923)
  arc A135 (41.0511, 85.923) -> (38.886, 84.673) centre (41.0511, 83.423) ccw
  line L102 (38.886, 84.673) -> (35.3294, 78.5128)
  arc A136 (35.3294, 78.5128) -> (35.3294, 76.0128) centre (37.4944, 77.2628) ccw
  line L103 (35.3294, 76.0128) -> (38.886, 69.8525)
  arc A137 (38.886, 69.8525) -> (41.0511, 68.6025) centre (41.0511, 71.1025) ccw
  line L104 (41.0511, 68.6025) -> (48.1643, 68.6025)
  arc A138 (48.1643, 68.6025) -> (50.3294, 69.8525) centre (48.1643, 71.1025) ccw
  line L105 (53.886, 78.5128) -> (50.3294, 84.673)
  arc A139 (53.886, 76.0128) -> (53.886, 78.5128) centre (51.7209, 77.2628) ccw
  line L106 (50.3294, 69.8525) -> (53.886, 76.0128)
  arc A140 (-48.1643, 85.923) -> (-50.3294, 84.673) centre (-48.1643, 83.423) ccw
  line L107 (-50.3294, 84.673) -> (-53.886, 78.5128)
  arc A141 (-53.886, 78.5128) -> (-53.886, 76.0128) centre (-51.7209, 77.2628) ccw
  line L108 (-53.886, 76.0128) -> (-50.3294, 69.8525)
  arc A142 (-50.3294, 69.8525) -> (-48.1643, 68.6025) centre (-48.1643, 71.1025) ccw
  line L109 (-48.1643, 68.6025) -> (-41.0511, 68.6025)
  arc A143 (-41.0511, 68.6025) -> (-38.886, 69.8525) centre (-41.0511, 71.1025) ccw
  line L110 (-38.886, 69.8525) -> (-35.3294, 76.0128)
  arc A144 (-35.3294, 76.0128) -> (-35.3294, 78.5128) centre (-37.4944, 77.2628) ccw
  line L111 (-41.0511, 85.923) -> (-48.1643, 85.923)
  arc A145 (-38.886, 84.673) -> (-41.0511, 85.923) centre (-41.0511, 83.423) ccw
  line L112 (-35.3294, 78.5128) -> (-38.886, 84.673)
  circle A146 centre (-0.25, 75.9996) radius 2.85
  point P0 (-79.2154, 0)
  point P1 (-98.9654, 0)
  point P2 (-89.2154, 0)
  point P3 (-39.6077, -68.6025)
  point P4 (-49.6077, -85.923)
  point P5 (-44.6077, -77.2628)
  point P6 (39.6077, -68.6025)
  point P7 (49.6077, -85.923)
  point P8 (44.6077, -77.2628)
  point P9 (79.2154, 0)
  point P10 (99.2154, 0)
  point P11 (89.2154, 0)
  point P12 (39.6077, 68.6025)
  point P13 (49.6077, 85.923)
  point P14 (44.6077, 77.2628)
  point P15 (-39.6077, 68.6025)
  point P16 (-49.6077, 85.923)
  point P17 (-44.6077, 77.2628)
  dimension "d112" = 25
  dimension "d115" = 4.7
  dimension "d118" = 3.5
  dimension "d124" = 3
  dimension "d159" = 0.5
  dimension "d161" = 360
  constraint coincident L8.start A89.centre
  constraint midpoint A7 L8.end
  constraint coincident L8 P2
  constraint coincident P2 A12.centre
  constraint concentric A12 A88
  constraint tangent L76 A95
  constraint tangent L73 A92
  constraint tangent A94 L76
  constraint tangent L71 A90
  constraint tangent L75 A94
  constraint tangent L71 A95
  constraint tangent A90 L72
  constraint tangent L74 A93
  constraint tangent A93 L75
  constraint tangent A91 L73
  constraint tangent L72 A91
  constraint tangent A92 L74
  measures "d112" distance of L8.end P1
  measures "d115" diameter of A12
  measures "d118" diameter of A88
  measures "d124" diameter of A89
extrude "Extrude16" add sketch "Sketch6" along normal blind 5 separate body contours A12 | L71 A90 L72 A91 L73 A92 L74 A93 L75 A94 L76 A95 makes body 3
extrude "Extrude17" cut sketch "Sketch6" against normal blind 4.2 contours A12 | A20 | A35 | A50 | A65 | A80 | A88 bodies 1
chamfer "Chamfer3" distance 1.5 angle 45 1 edges at (-90.847, -0.6328, -5) on bodies 3